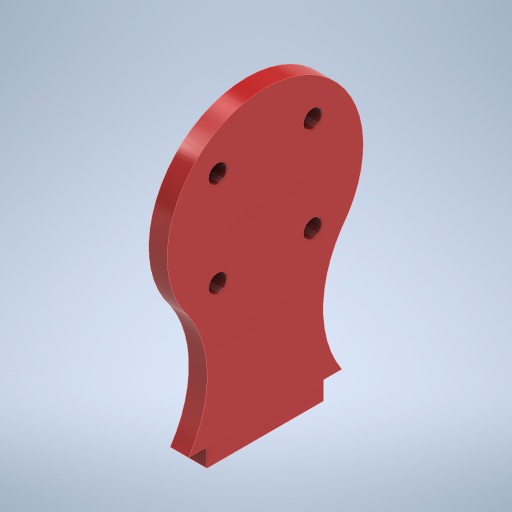
# Autodesk Inventor part: soporteEncoder
Saved by Autodesk Inventor 2024.3 (Build 283343000, 343)
## iProperties
Created: 2024-05-25
Part Number: soporteEncoder
Material: PMMA Plastic
Document SubType Name: Modeling
Designer: USUARIO
Density: 1.188 g/cm^3
Appearance: Red
Author: USUARIO
Autodesk Inventor part; units mm, degrees
ref_plane "YZ Plane" through (0, 0, 0) normal (1, 0, 0) x (0, 1, 0)
ref_plane "XZ Plane" through (0, 0, 0) normal (0, 1, 0) x (-1, 0, 0)
ref_plane "XY Plane" through (0, 0, 0) normal (0, 0, 1) x (1, 0, 0)
sketch "Sketch1" plane through (0, 0, 0) normal (1, 0, 0) x (0, 1, 0)
  line L0 (0, 0) -> (3, 0)
  line L1 (3, 0) -> (3, -19) construction
  line L2 (3, -19) -> (0, -19)
  line L3 (0, -19) -> (0, 0)
  line L4 (3, 0) -> (3, 3) construction
  line L5 (3, 3) -> (23.0125, 3) construction
  line L6 (33, 3) -> (33, -22) construction
  line L7 (33, -22) -> (23.0125, -22) construction
  line L8 (3, -22) -> (3, -19)
  line L9 (33, -9.5) -> (40.75, -9.5) construction
  line L10 (40.75, -9.5) -> (40.75, -17.25) construction
  line L11 (40.75, -17.25) -> (33, -17.25) construction
  line L12 (33, -17.25) -> (33, -9.5) construction
  circle A0 centre (40.75, -17.25) radius 1.5
  line L13 (40.75, -17.25) -> (25.25, -17.25) construction
  line L14 (25.25, -17.25) -> (25.25, -1.75) construction
  line L15 (25.25, -1.75) -> (40.75, -1.75) construction
  line L16 (40.75, -1.75) -> (40.75, -17.25) construction
  circle A1 centre (25.25, -17.25) radius 1.5
  circle A2 centre (25.25, -1.75) radius 1.5
  circle A3 centre (40.75, -1.75) radius 1.5
  arc A4 (23.0125, -22) -> (23.0125, 3) centre (33, -9.5) ccw
  line L17 (23.0125, 3) -> (33, 3) construction
  line L18 (23.0125, -22) -> (3, -22) construction
  arc A5 (3, 3) -> (23.0125, 3) centre (13.0063, 17.9624) ccw
  arc A6 (23.0125, -22) -> (3, -22) centre (13.0063, -36.9624) ccw
  line L19 (3, 0) -> (3, 3)
  line L20 (3, -19) -> (3, 0) construction
  arc A7 (23.0125, 3) -> (23.0125, -22) centre (33, -9.5) ccw construction
  point P0 (23.0125, -22)
  point P1 (23.0125, 3)
  dimension "d0" = 3
  dimension "d1" = 19
  dimension "d2" = 3
  dimension "d3" = 30
  dimension "d4" = 25
  dimension "d5" = 7.75
  dimension "d6" = 7.75
  dimension "d7" = 3
  dimension "d8" = 15.5
  dimension "d9" = 15.5
  dimension "d10" = 3
  dimension "d11" = 3
  dimension "d12" = 3
  dimension "d13" = 32
  dimension "d16" = 18
  dimension "d17" = 18
  constraints: 42 end point, 13 parallel, 8 centre point, 8 point on circle, 5 coincident, 5 horizontal, 5 perpendicular, 1 midpoint, 1 vertical
  measures "d0" distance of L1.end L2.end
  measures "d1" distance of L0.end L1.end
  measures "d2" distance of L0.end L4.end
  measures "d3" distance of L6.end L8.start
  measures "d4" distance of L6.start L6.end
  measures "d5" distance of L10.end L11.end
  measures "d6" distance of L9.end L10.end
  measures "d7" diameter of A0
  measures "d8" distance of L14.end L15.end
  measures "d9" distance of L13.end L14.end
  measures "d10" diameter of A1
  measures "d11" diameter of A2
  measures "d12" diameter of A3
  measures "d13" diameter of A4
  measures "d16" radius of A5
  measures "d17" radius of A6
extrude "Extrusion1" add sketch "Sketch1" along normal blind 3
body "Solid1"
